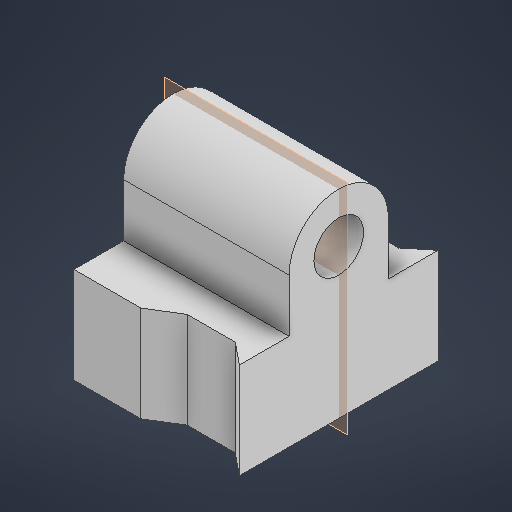
# Autodesk Inventor part: Peça2
Saved by Autodesk Inventor 2027.1 (Build 311270010, 270A)
## iProperties
Created: 2026-09-24
Part Number: Peça2
Material: Genérico
Document SubType Name: Modeling
Designer: carlo
Density: 1 g/cm^3
Appearance: Padrão
Author: carlo
Autodesk Inventor part; units mm, degrees
ref_plane "YZ Plane" through (0, 0, 0) normal (1, 0, 0) x (0, 1, 0)
ref_plane "XZ Plane" through (0, 0, 0) normal (0, 1, 0) x (-1, 0, 0)
sketch "Esboço1" plane through (0, 0, 0) normal (0, 1, 0) x (-1, 0, 0)
  line L0 (25, 30) -> (-25, 30)
  line L1 (-25, 30) -> (-25, -30)
  line L2 (-25, -30) -> (25, -30)
  line L3 (25, -30) -> (25, 30)
  line L4 (25, 30) -> (-25, -30) construction
  line L5 (-25, 30) -> (25, -30) construction
  point P0 (0, 0)
  dimension "d0" = 50
  dimension "d1" = 60
  constraints: 12 end point, 2 midpoint, 2 parallel, 1 horizontal, 1 perpendicular
  measures "d0" distance of L2.end L1.end
  measures "d1" distance of L1.end L0.end
extrude "Extrusão1" add sketch "Esboço1" along normal blind 60
sketch "Esboço2" plane through (25, 0, 30) normal (1, 0, 0) x (0, 0, -1)
  line L0 (0, 60) -> (15, 60)
  line L1 (15, 60) -> (15, 28.9851)
  line L2 (15, 28.9851) -> (0, 28.9851)
  line L3 (0, 28.9851) -> (0, 60)
  line L4 (0, 60) -> (60, 60) projected
  line L5 (60, 60) -> (45, 60)
  line L6 (45, 60) -> (45, 28.9851)
  line L7 (45, 28.9851) -> (60, 28.9851)
  line L8 (60, 28.9851) -> (60, 60)
  point P0 (30, 0)
  dimension "d4" = 15
  dimension "d5" = 15
  constraints: 16 end point, 4 parallel, 2 collinear, 2 perpendicular, 2 point on line
  measures "d4" distance between parallel lines of L1 L3
  measures "d5" distance between parallel lines of L6 L8
extrude "Extrusão2" cut sketch "Esboço2" against normal blind 60
fillet "Arredondamento1" radius 15 2 edges at (0, 60, 15) (0, 60, -15)
sketch "Esboço3" plane through (25, 0, 30) normal (1, 0, 0) x (0, 0, -1)
  arc A0 (45, 45) -> (15, 45) centre (30, 45) ccw projected
  point P0 (30, 0)
  constraints: 1 coincident
hole "Furo1" at (25, 45, 0) direction (-1, 0, 0) diameter 15 end through all
sketch "Esboço4" plane through (25, 28.9851, 30) normal (0, 1, 0) x (1, 0, 0)
  line L0 (0, 0) -> (-50, 0) projected
  line L1 (-50, 0) -> (-29.7763, 0)
  line L2 (-21.1397, 5.3332) -> (-6.6144, 5.3332)
  line L3 (-6.6144, 5.3332) -> (0, 0)
  line L4 (0, 0) -> (-34.3564, 0)
  line L5 (-21.1397, 5.3332) -> (-29.7763, 0)
  point P0 (-25, 30)
  constraints: 10 end point, 2 point on line, 1 horizontal
extrude "Extrusão3" cut sketch "Esboço4" against normal blind 60
mirror "Espelhar1" about plane through (0, 0, 0) normal (0, 0, 1) of "Extrusão3"
